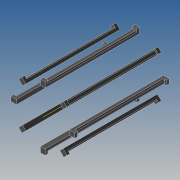
# Autodesk Inventor part: 1402_Bias Coil Spacer_V1
Saved by Autodesk Inventor 2020 (Build 240168000, 168)
## iProperties
Created: 2019-11-11
Part Number: 1402_Bias Coil Spacer_V1
Material: ABS Plastic
Document SubType Name: Modeling
Designer: RFLab
Density: 1.06 g/cm^3
Appearance: Smooth - White
Author: RFLab
Autodesk Inventor part; units mm, degrees
ref_plane "YZ Plane" through (0, 0, 0) normal (1, 0, 0) x (0, 1, 0)
ref_plane "XZ Plane" through (0, 0, 0) normal (0, 1, 0) x (-1, 0, 0)
ref_plane "XY Plane" through (0, 0, 0) normal (0, 0, 1) x (1, 0, 0)
sketch "Sketch1" plane through (0, 0, 0) normal (0, 0, 1) x (1, 0, 0)
  line L0 (-2.5, 3) -> (2.5, 3)
  line L1 (2.5, 3) -> (2.5, -3)
  line L2 (2.5, -3) -> (-2.5, -3)
  line L3 (-2.5, -3) -> (-2.5, 3)
  point P0 (0, 0)
  dimension "d0" = 5
  dimension "d1" = 6
  dimension "d2" = 3
  dimension "d3" = 2.5
  constraints: 8 end point, 2 parallel, 1 horizontal, 1 perpendicular
  measures "d0" distance of L0.start L0.end
  measures "d1" distance of L0.end L1.end
  measures "d2" distance from line of L0 point (0, 0)
  measures "d3" distance from line of point (0, 0) L1
extrude "Extrusion1" add sketch "Sketch1" along normal blind 102
sketch "Sketch2" plane through (2.5, -3, 0) normal (1, 0, 0) x (0, 0, -1)
  line L0 (0, 6) -> (-102, 6) projected
  line L1 (-99, 6) -> (-3, 6)
  line L2 (-3, 6) -> (-3, 4)
  line L3 (-3, 4) -> (-99, 4)
  line L4 (-99, 4) -> (-99, 6)
  point P0 (0, 3)
  point P1 (-3, 6)
  dimension "d6" = 3
  dimension "d7" = 96
  dimension "d8" = 2
  constraints: 8 end point, 2 parallel, 1 horizontal, 1 perpendicular, 1 point on line
  measures "d6" distance of L1.end L0.start
  measures "d7" distance of L1.start L1.end
  measures "d8" distance of L3.end L1.start
extrude "Extrusion2" cut sketch "Sketch2" against normal through all
fillet "Fillet1" radius 1 2 edges at (2.5, 1, 51) (-2.5, 1, 51)
sketch3d "3D Sketch1"
pattern_circular "Circular Pattern1" count 8 over 360 about axis through (0, -31.525, 102) along (0, 0, -1) of "Extrusion1", "Extrusion2", "Fillet1"
sketch "Sketch3" plane through (0, 0, 0) normal (0, 0, 1) x (1, 0, 0)
  line L0 (0, 0) -> (0, -31.525)
  line L1 (-2.5, -66.05) -> (2.5, -66.05) projected
  line L2 (2.5, 3) -> (-2.5, 3) projected
  dimension "d17" = 69.05
  dimension "d18" = 3
  dimension "d19" = 31.525
  constraints: 2 end point, 1 vertical
  measures "d17" distance between parallel lines of L1 L2
  measures "d18" distance from line of L2 L0.start
  measures "d19" distance of L0.start L0.end
equation "\"d2\" = 0.5 * d1"
equation "\"d3\" = 0.5 * d0"
equation "\"d19\" = 0.5 * d17 - d18"
body "Solid1"
